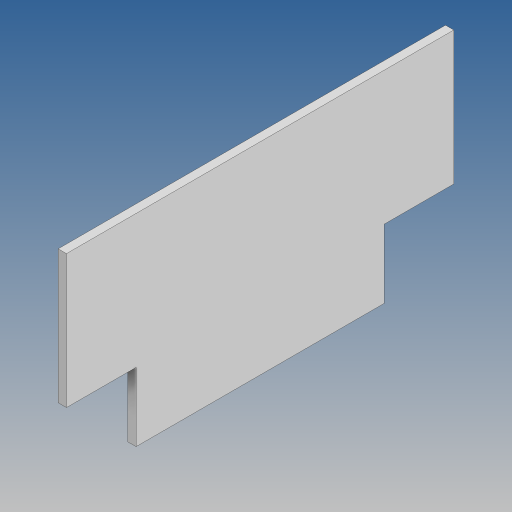
# Autodesk Inventor part: Pieza10
Saved by Autodesk Inventor 2024 (Build 280153000, 153)
## iProperties
Created: 2024-05-31
Part Number: Pieza10
Material: Genérico
Document SubType Name: Modeling
Designer: Pablo
Density: 1 g/cm^3
Appearance: Valor por defecto
Author: Pablo
Autodesk Inventor part; units mm, degrees
ref_plane "YZ Plane" through (0, 0, 0) normal (1, 0, 0) x (0, 1, 0)
ref_plane "XZ Plane" through (0, 0, 0) normal (0, 1, 0) x (-1, 0, 0)
ref_plane "XY Plane" through (0, 0, 0) normal (0, 0, 1) x (1, 0, 0)
sketch "Boceto1" plane through (0, 0, 0) normal (1, 0, 0) x (0, 1, 0)
  line L0 (0, 0) -> (24.8, 0)
  line L1 (24.8, 0) -> (24.8, -89.7)
  line L2 (24.8, -89.7) -> (0, -89.7)
  line L3 (0, -89.7) -> (0, 0)
  line L4 (0, -44.85) -> (73, -44.85) construction
  line L5 (24.8, -44.85) -> (73, -44.85) construction
  line L6 (24.8, 25.15) -> (73, 25.15)
  line L7 (73, 25.15) -> (73, -114.85)
  line L8 (73, -114.85) -> (24.8, -114.85)
  line L9 (24.8, -114.85) -> (24.8, 25.15)
  line L10 (24.8, 25.15) -> (73, -114.85) construction
  line L11 (73, 25.15) -> (24.8, -114.85) construction
  point P0 (48.9, -44.85)
  dimension "d0" = 24.8
  dimension "d1" = 89.7
  dimension "d2" = 73
  dimension "d3" = 140
  constraints: 24 end point, 5 midpoint, 5 parallel, 2 horizontal, 2 perpendicular, 1 collinear, 1 point on line
  measures "d0" distance of L1.end L2.end
  measures "d1" distance of L0.end L1.end
  measures "d2" distance of L4.start L4.end
  measures "d3" distance of L6.end L7.end
extrude "Extrusión1" add sketch "Boceto1" along normal blind 3
